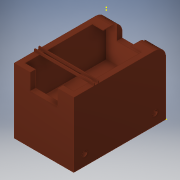
# Autodesk Inventor part: Design
Saved by Autodesk Inventor 2018 (Build 220112000, 112)
## iProperties
Created: 2018-01-20
Part Number: Design
Material: Copper
Document SubType Name: Modeling
Designer: abdul
Density: 8.94 g/cm^3
Appearance: Copper - Satin
Author: abdul
Autodesk Inventor part; units mm, degrees
ref_plane "YZ Plane" through (0, 0, 0) normal (1, 0, 0) x (0, 1, 0)
ref_plane "XZ Plane" through (0, 0, 0) normal (0, 1, 0) x (-1, 0, 0)
ref_plane "XY Plane" through (0, 0, 0) normal (0, 0, 1) x (1, 0, 0)
sketch "Sketch10" plane through (0, 0, 0) normal (0, 1, 0) x (-1, 0, 0)
  point P0 (0, 0)
sketch "Sketch11" plane through (0, 0, 0) normal (0, 0, 1) x (1, 0, 0)
  point P0 (0, 0)
sketch "Sketch12" plane through (0, 0, 0) normal (0, 0, 1) x (1, 0, 0)
  line L0 (0, 0) -> (1100, 0)
  line L1 (1100, 0) -> (1100, 1200)
  line L2 (1100, 1200) -> (0, 1200)
  line L3 (0, 1200) -> (0, 0)
  dimension "d20" = 1100
  dimension "d21" = 1200
  constraints: 8 end point, 2 parallel, 1 horizontal, 1 perpendicular
  measures "d20" distance of L2.end L1.end
  measures "d21" distance of L1.end L0.end
extrude "Extrusion6" add sketch "Sketch12" along normal blind 1700
sketch "Sketch13" plane through (1100, 0, 0) normal (1, 0, 0) x (0, 0, -1)
  line L0 (-100, 100) -> (-1600, 100)
  line L1 (-1600, 100) -> (-1600, 1200)
  line L2 (-1600, 1200) -> (-100, 1200)
  line L3 (-100, 1200) -> (-100, 100)
  point P0 (0, 0)
  dimension "d24" = 1500
  constraints: 8 end point, 2 parallel, 1 horizontal, 1 perpendicular
  measures "d24" distance of L1.end L2.end
extrude "Extrusion7" cut sketch "Sketch13" against normal blind 1000
sketch "Sketch16" plane through (100, 0, 0) normal (1, 0, 0) x (0, 0, -1)
  circle A0 centre (-1499, 200) radius 50
  circle A1 centre (-201, 200) radius 50
  point P0 (0, 0)
  dimension "d34" = 100
  dimension "d35" = 100
  constraints: 2 centre point
  measures "d34" diameter of A0
  measures "d35" diameter of A1
extrude "Extrusion10" cut sketch "Sketch16" along normal blind 1200 and the other way blind 200
sketch "Sketch18" plane through (1100, 100, 100) normal (0, 0, 1) x (1, 0, 0)
  line L0 (0, 0) -> (-1000, 0) projected
  line L1 (-1000, 1100) -> (0, 1100) projected
  line L2 (0, 0) -> (-100, 0)
  line L3 (-100, 0) -> (-100, 1100)
  line L4 (-100, 1100) -> (0, 1100)
  line L5 (0, 1100) -> (0, 0)
  point P0 (-1100, -100)
  dimension "d43" = 100
  constraints: 8 end point, 2 parallel, 1 horizontal, 1 perpendicular, 1 point on line
  measures "d43" distance of L3.end L4.end
extrude "Extrusion12" add sketch "Sketch18" along normal blind 1500
sketch "Sketch19" plane through (0, 0, 1700) normal (0, 0, 1) x (1, 0, 0)
  line L0 (100, 500) -> (1000, 500)
  line L1 (1000, 500) -> (1000, 510)
  line L2 (1000, 510) -> (100, 510)
  line L3 (100, 510) -> (100, 500)
  point P0 (0, 0)
  dimension "d46" = 900
  dimension "d47" = 10
  constraints: 8 end point, 2 parallel, 1 horizontal, 1 perpendicular
  measures "d46" distance of L2.end L1.end
  measures "d47" distance of L1.end L0.end
extrude "Extrusion13" add sketch "Sketch19" against normal blind 1700
sketch "Sketch20" plane through (0, 0, 0) normal (0, 0, -1) x (-1, 0, 0)
  line L0 (-805, 1200) -> (-295, 1200)
  line L1 (-295, 1200) -> (-295, 900)
  line L2 (-295, 900) -> (-805, 900)
  line L3 (-805, 900) -> (-805, 1200)
  point P0 (0, 0)
  dimension "d58" = 510
  dimension "d59" = 300
  constraints: 8 end point, 2 parallel, 1 horizontal, 1 perpendicular
  measures "d58" distance of L1.end L2.end
  measures "d59" distance of L0.end L1.end
extrude "Extrusion14" cut sketch "Sketch20" against normal blind 1700
sketch "Sketch21" plane through (1100, 1200, 1700) normal (0, 1, 0) x (1, 0, 0)
  line L0 (0, 1700) -> (0, 0) projected
  line L1 (-1100, 1700) -> (-1100, 0) projected
  line L2 (0, 470.5254) -> (-1100, 470.5254)
  line L3 (-1100, 470.5254) -> (-1100, 370.5254)
  line L4 (-1100, 370.5254) -> (0, 370.5254)
  line L5 (0, 370.5254) -> (0, 470.5254)
  dimension "d60" = 100
  constraints: 8 end point, 2 parallel, 2 point on line, 1 horizontal, 1 perpendicular
  measures "d60" distance of L3.end L2.end
extrude "Extrusion15" add sketch "Sketch21" along normal blind 40
sketch "Sketch22" plane through (1100, 1240, 1700) normal (0, 1, 0) x (1, 0, 0)
  line L0 (-1100, 470.5254) -> (-1100, 370.5254) projected
  line L1 (0, 370.5254) -> (0, 470.5254) projected
  line L2 (-1100, 450.525) -> (0, 450.525)
  line L3 (0, 450.525) -> (0, 390.525)
  line L4 (0, 390.525) -> (-1100, 390.525)
  line L5 (-1100, 390.525) -> (-1100, 450.525)
  point P0 (-1100, 1700)
  dimension "d63" = 60
  constraints: 8 end point, 2 parallel, 2 point on line, 1 horizontal, 1 perpendicular
  measures "d63" distance of L2.end L3.end
extrude "Extrusion16" cut sketch "Sketch22" against normal blind 40
sketch "Sketch23" plane through (1100, 1240, 1700) normal (0, 1, 0) x (1, 0, 0)
  point P0 (-1100, 1700)
sketch "Sketch25" plane through (1100, 0, 0) normal (1, 0, 0) x (0, 0, -1)
  point P0 (0, 0)
sketch "Sketch27" plane through (0, 0, 0) normal (0, 0, -1) x (-1, 0, 0)
  line L0 (-865, 700) -> (-785, 700)
  line L1 (-785, 700) -> (-785, 600)
  line L2 (-785, 600) -> (-865, 600)
  line L3 (-865, 600) -> (-865, 700)
  line L4 (0, 0) -> (-1100, 0) projected
  line L5 (-1100, 0) -> (-1100, 1200) projected
  line L6 (-805, 900) -> (-805, 1200) projected
  line L7 (-315, 700) -> (-235, 700)
  line L8 (-235, 700) -> (-235, 600)
  line L9 (-235, 600) -> (-315, 600)
  line L10 (-315, 600) -> (-315, 700)
  line L11 (-295, 1200) -> (-295, 900) projected
  dimension "d77" = 100
  dimension "d78" = 80
  dimension "d79" = 600
  dimension "d81" = 20
  dimension "d82" = 100
  dimension "d83" = 80
  dimension "d84" = 600
  dimension "d85" = 20
  constraints: 16 end point, 4 parallel, 2 horizontal, 2 perpendicular
  measures "d77" distance of L2.end L0.start
  measures "d78" distance of L1.end L2.end
  measures "d79" distance between parallel lines of L4 L2
  measures "d81" distance between parallel lines of L1 L6
  measures "d82" distance of L9.end L7.start
  measures "d83" distance of L8.end L9.end
  measures "d84" distance between parallel lines of L4 L9
  measures "d85" distance between parallel lines of L11 L10
extrude "Extrusion17" cut sketch "Sketch27" against normal blind 10
sketch "Sketch28" plane through (0, 1200, 1229.4746) normal (0, 1, 0) x (1, 0, 0)
  line L0 (100, 0) -> (100, 1129.4746) projected
  line L1 (295, 1129.4746) -> (100, 1129.4746)
  line L2 (100, 1129.4746) -> (100, 878.7986)
  line L3 (100, 878.7986) -> (295, 878.7986)
  line L4 (295, 878.7986) -> (295, 1129.4746)
  point P0 (0, 1229.4746)
  point P1 (100, 1029.4746)
  dimension "d90" = 250.676
  constraints: 8 end point, 2 parallel, 1 horizontal, 1 perpendicular, 1 point on line
  measures "d90" distance of L2.end L0.end
extrude "Extrusion18" add sketch "Sketch28" against normal blind 10
sketch "Sketch29" plane through (805, 1200, 0) normal (0, 1, 0) x (1, 0, 0)
  line L0 (0, 0) -> (0, -100) projected
  line L1 (195, -100) -> (195, -1229.4746) projected
  line L2 (0, -100) -> (195, -100)
  line L3 (195, -100) -> (195, -350.676)
  line L4 (195, -350.676) -> (0, -350.676)
  line L5 (0, -350.676) -> (0, -100)
  point P0 (-805, 0)
  dimension "d93" = 250.676
  constraints: 8 end point, 2 parallel, 1 horizontal, 1 perpendicular, 1 point on line
  measures "d93" distance of L2.end L3.end
extrude "Extrusion19" add sketch "Sketch29" against normal blind 10
sketch "Sketch30" plane through (0, 1200, 0) normal (0, 1, 0) x (1, 0, 0)
  point P0 (0, 0)
fillet "Fillet3" radius 200 2 edges at (952.5, 1200, 0) (147.5, 1200, 0)
sketch "Sketch31" plane through (0, 0, 1700) normal (-1, 0, 0) x (0, 0, 1)
  circle A0 centre (-1499, 200) radius 50 projected
  circle A1 centre (-1499, 200) radius 50
  point P0 (-1700, 0)
  constraints: 1 centre point, 1 coincident
extrude "Extrusion20" cut sketch "Sketch31" against normal blind 10000
sketch "Sketch32" plane through (0, 0, 1700) normal (-1, 0, 0) x (0, 0, 1)
  circle A0 centre (-201, 200) radius 50 projected
  circle A1 centre (-201, 200) radius 50
  point P0 (-1700, 0)
  constraints: 1 centre point, 1 coincident, 1 concentric
extrude "Extrusion21" cut sketch "Sketch32" against normal blind 10000
body "Solid2"
